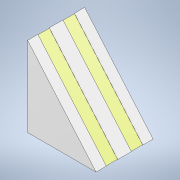
# Autodesk Inventor part: 三明治
Saved by Autodesk Inventor 2022 (Build 260153000, 153)
## iProperties
Created: 2023-03-16
Part Number: 三明治
Material: 一般
Document SubType Name: Modeling
Designer: User
Mass: 104.557 g
Surface Area: 153.749 cm^2
Volume: 104.557 cm^3
Density: 1 g/cm^3
Appearance: 預設
Author: User
Autodesk Inventor part; units mm, degrees
ref_plane "YZ Plane" through (0, 0, 0) normal (1, 0, 0) x (0, 1, 0)
ref_plane "XZ Plane" through (0, 0, 0) normal (0, 1, 0) x (-1, 0, 0)
sketch "草圖1" plane through (0, 0, 0) normal (0, 0, 1) x (1, 0, 0)
  line L0 (-12, 0) -> (72, 0) construction
  line L1 (0, -14) -> (0, 84) construction
  line L2 (0, 0) -> (60, 0)
  line L3 (0, 70) -> (0, 0)
  line L4 (0, 70) -> (60, 0)
  dimension "d0" = 60
  dimension "d1" = 70
  constraints: 6 end point, 2 point on line, 1 horizontal
  measures "d0" distance from line of L1 L2.end
  measures "d1" distance from line of L0 L3.start
extrude "擠出1" add sketch "草圖1" along normal mid plane 50
ref_plane "工作平面1" through (0, 0, 2) normal (0, 0, 1) x (1, 0, 0)
ref_plane "工作平面2" through (0, 0, 6) normal (0, 0, 1) x (1, 0, 0)
sketch "草圖3" plane through (0, 0, 6) normal (0, 0, 1) x (1, 0, 0)
  line L0 (0, 0) -> (0, 70) construction
  line L1 (0, 70) -> (60, 0) construction
  line L2 (60, 0) -> (0, 0) projected
  line L3 (59.7826, 0.1) -> (0.1, 69.7297)
  line L4 (0.1, 69.7297) -> (0.1, 0.1)
  line L5 (0.1, 0.1) -> (59.7826, 0.1)
  line L6 (0, 0) -> (0, 70) projected
  line L7 (0, 70) -> (60, 0) projected
  line L8 (60, 0) -> (0, 0) projected
  dimension "d7" = 0.1
  constraints: 6 end point, 2 other
  measures "d7" distance between parallel lines of L1 L3
extrude "擠出2" cut sketch "草圖3" along normal blind 10
mirror "鏡射1" about plane through (0, 0, 0) normal (0, 0, 1) of "擠出2"
